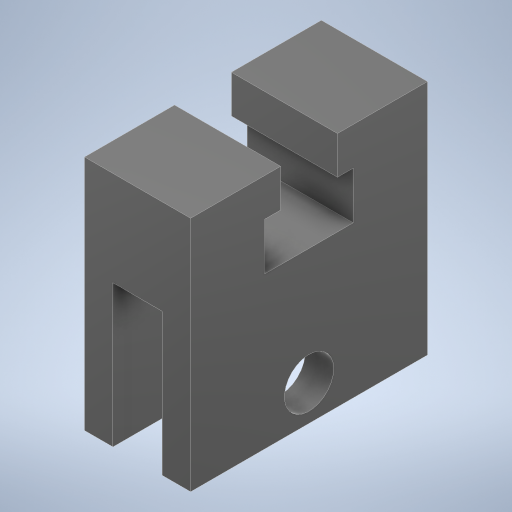
# Autodesk Inventor part: RollYAxisEnd
Saved by Autodesk Inventor 2023 (Build 270158000, 158)
## iProperties
Created: 2023-10-26
Part Number: RollYAxisEnd
Material: Thermoplastic Resin
Document SubType Name: Modeling
Designer: Mustapha
Density: 1.28 g/cm^3
Appearance: Smooth - Black
Mass: 5.28694 g
Surface Area: 31.1216 cm^2
Volume: 4.13042 cm^3
Author: Mustapha
Autodesk Inventor part; units mm, degrees
ref_plane "YZ Plane" through (0, 0, 0) normal (1, 0, 0) x (0, 1, 0)
ref_plane "XZ Plane" through (0, 0, 0) normal (0, 1, 0) x (-1, 0, 0)
ref_plane "XY Plane" through (0, 0, 0) normal (0, 0, 1) x (1, 0, 0)
sketch "Sketch1" plane through (0, 0, 0) normal (0, 1, 0) x (-1, 0, 0)
  line L0 (0, 0) -> (3, 0)
  line L1 (3, 0) -> (3, -25)
  line L2 (3, -25) -> (0, -25)
  line L3 (0, -25) -> (0, 0)
  line L4 (8.2, 0) -> (11.2, 0)
  line L5 (11.2, 0) -> (11.2, -25)
  line L6 (11.2, -25) -> (8.2, -25)
  line L7 (8.2, -25) -> (8.2, 0)
  point P0 (0, -12.5)
  point P1 (8.2, -12.5)
  dimension "d0" = 25
  dimension "d1" = 3
  dimension "d2" = 25
  dimension "d3" = 3
  dimension "d4" = 5.2
  constraints: 16 end point, 4 parallel, 2 horizontal, 2 midpoint, 2 perpendicular
  measures "d0" distance between parallel lines of L2 L0
  measures "d1" distance from line of point (0, -12.5) L1
  measures "d2" distance between parallel lines of L6 L4
  measures "d3" distance from line of point (8.2, -12.5) L5
  measures "d4" distance between parallel lines of L1 L7
extrude "Extrusion1" add sketch "Sketch1" along normal blind 15
sketch "Sketch2" plane through (0, 15, 0) normal (0, 1, 0) x (1, 0, 0)
  line L0 (-11.2, 25) -> (-11.2, 0) projected
  line L1 (-11.2, 0) -> (0, 0)
  line L2 (0, 0) -> (0, 25)
  line L3 (0, 25) -> (-11.2, 25)
  line L4 (-11.2, 25) -> (-11.2, 0)
  point P0 (0, 0)
  constraints: 8 end point, 2 parallel, 1 horizontal, 1 perpendicular
extrude "Extrusion2" add sketch "Sketch2" along normal blind 10
sketch "Sketch3" plane through (0, 0, 0) normal (1, 0, 0) x (0, 0, -1)
  line L0 (0, 25) -> (25, 25) projected
  line L1 (12.5, 25) -> (12.5, 0.2306)
  line L2 (9.5, 25) -> (9.5, 21)
  line L3 (9.5, 21) -> (7.8272, 21)
  line L4 (7.8272, 21) -> (7.8272, 16)
  line L5 (7.8272, 16) -> (12.5, 16)
  line L6 (15.5, 25) -> (15.5, 21)
  line L7 (15.5, 21) -> (17.1728, 21)
  line L8 (17.1728, 21) -> (17.1728, 16)
  line L9 (17.1728, 16) -> (12.5, 16)
  line L10 (9.5, 25) -> (15.5, 25)
  circle A0 centre (12.5, 3.7087) radius 2.6
  point P0 (0, 0)
  point P1 (8.6636, 21)
  dimension "d9" = 6
  dimension "d10" = 5
  dimension "d11" = 8
  dimension "d14" = 5.2
  constraints: 20 end point, 4 symmetric about line, 3 perpendicular, 3 point on line, 2 midpoint, 2 vertical, 1 centre point, 1 collinear
  measures "d9" diameter of L2 L1
  measures "d10" distance from line of L5 point (8.664, 21)
  measures "d11" diameter of point (8.664, 21) L0
  measures "d14" diameter of A0
extrude "Extrusion3" cut sketch "Sketch3" against normal blind 20
body "Solid1"
